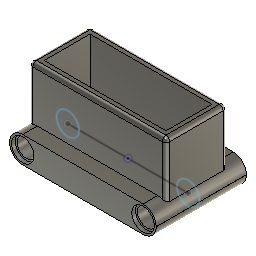
Servo_mount (Autodesk Fusion 360 design; units mm, degrees)
Autodesk Fusion 360 part; units mm, degrees
note: some values were not read from the file. Set by a fixed rule: which face or edge a step refers to.
sketch "Sketch1" plane through (0, 0, 0) normal (0, 1, 0) x (1, 0, 0)
  circle A0 centre (-16, 0) radius 2.5
  circle A1 centre (16, 0) radius 2.5
  line L0 (16.01, -3.5) -> (-16.01, -3.5)
  line L1 (-19.5, -0.01) -> (-19.5, 0.01)
  line L2 (-16.01, 3.5) -> (16.01, 3.5)
  line L3 (19.5, 0.01) -> (19.5, -0.01)
  arc A2 (-16.01, 3.5) -> (-19.5, 0.01) centre (-16.01, 0.01) ccw
  arc A3 (-19.5, -0.01) -> (-16.01, -3.5) centre (-16.01, -0.01) ccw
  arc A4 (19.5, 0.01) -> (16.01, 3.5) centre (16.01, 0.01) ccw
  arc A5 (16.01, -3.5) -> (19.5, -0.01) centre (16.01, -0.01) ccw
  line L4 (-13.5, 0) -> (-16, 0)
  circle A6 centre (16.01, 0.01) radius 3
  circle A7 centre (-16, 0) radius 3
  dimension "d7" = 5
  dimension "d9" = 5
  dimension "d12" = 3.49
  dimension "d13" = 3.49
  dimension "d14" = 3.49
  dimension "d15" = 3.49
  dimension "d53" = 6
  dimension "d54" = 6
  constraint coincident A0.centre L4.end
  constraint horizontal L0
  constraint perpendicular L0 L1
  constraint parallel L0 L2
  constraint parallel L1 L3
  constraint tangent L2 A2
  constraint tangent L1 A2
  constraint tangent L1 A3
  constraint tangent L0 A3
  constraint tangent L2 A4
  constraint tangent L3 A4
  constraint tangent L0 A5
  constraint tangent L3 A5
  constraint coincident A0 L4.start
  constraint concentric A4 A6
  measures "d7" diameter of A0
  measures "d9" diameter of A1
  measures "d12" radius of A2
  measures "d13" radius of A3
  measures "d14" radius of A4
  measures "d15" radius of A5
  measures "d53" diameter of A6
  measures "d54" diameter of A7
sketch "Sketch2" plane through (0, 0, 0) normal (0, 0, 1) x (1, 0, 0)
  line L0 (16.2, 6.1) -> (-16.2, 6.1)
  line L1 (-16.2, 6.1) -> (-16.2, -6.1)
  line L2 (-16.2, -6.1) -> (16.2, -6.1)
  line L3 (16.2, -6.1) -> (16.2, 6.1)
  line L4 (16.2, 6.1) -> (-16.2, -6.1) construction
  line L5 (-16.2, 6.1) -> (16.2, -6.1) construction
  line L6 (11.5, 6.1) -> (-11.5, 6.1)
  line L7 (-11.5, 6.1) -> (-11.5, -6.1)
  line L8 (-11.5, -6.1) -> (11.5, -6.1)
  line L9 (11.5, -6.1) -> (11.5, 6.1)
  line L10 (11.5, 6.1) -> (-11.5, -6.1) construction
  line L11 (-11.5, 6.1) -> (11.5, -6.1) construction
  line L12 (0, 0) -> (14, 0)
  line L13 (0, 0) -> (-14, 0)
  circle A0 centre (14, 0) radius 0.75
  circle A1 centre (-14, 0) radius 0.75
  line L14 (18.2, -8.1) -> (-18.2, -8.1)
  line L15 (-18.2, -8.1) -> (-18.2, 8.1)
  line L16 (-18.2, 8.1) -> (18.2, 8.1)
  line L17 (18.2, 8.1) -> (18.2, -8.1)
  line L18 (18.2, -8.1) -> (-18.2, 8.1) construction
  line L19 (-18.2, -8.1) -> (18.2, 8.1) construction
  dimension "d16" = 32.4
  dimension "d17" = 12.2
  dimension "d18" = 23
  dimension "d19" = 14
  dimension "d20" = 14
  dimension "d21" = 1.5
  dimension "d22" = 1.5
  dimension "d23" = 36.4
  dimension "d24" = 16.2
  constraint horizontal L0
  constraint perpendicular L0 L1
  constraint parallel L0 L2
  constraint parallel L1 L3
  constraint coincident L4 L12.start
  constraint coincident L5 L12.start
  constraint coincident L12.start L13.start
  constraint horizontal L6
  constraint perpendicular L6 L7
  constraint parallel L6 L8
  constraint parallel L7 L9
  constraint coincident L10 L12.start
  constraint coincident L11 L12.start
  constraint horizontal L12
  constraint horizontal L13
  constraint coincident L12.end A0.centre
  constraint coincident L13.end A1.centre
  constraint horizontal L14
  constraint perpendicular L14 L15
  constraint parallel L14 L16
  constraint parallel L15 L17
  constraint coincident L18 L12.start
  constraint coincident L19 L12.start
  measures "d16" distance of L1.end L2.end
  measures "d17" distance of L0.end L1.end
  measures "d18" distance of L7.end L8.end
  measures "d19" distance of L12.start L12.end
  measures "d20" distance of L12.start L13.end
  measures "d21" diameter of A0
  measures "d22" diameter of A1
  measures "d23" distance of L15.end L16.end
  measures "d24" distance of L14.end L15.end
extrude "Extrude1" add sketch "Sketch2" along normal blind 7 contours L14 L15 L16 L17
extrude "Extrude2" add sketch "Sketch2" along normal blind 4 contours L0 L2 L3 L9 | L0 L1 L2 L7
move_body "Move1" bodies 1 to x (1, 0, 0) y (0, 1, 0) z (0, 0, 1) at (0, 0, 0.5)
extrude "Extrude3" cut sketch "Sketch1" along normal blind 9 contours A0 | A1
extrude "Extrude4" cut sketch "Sketch1" against normal blind 10 contours A0 | A1
extrude "Extrude5" add sketch "Sketch1" along normal blind 12 contours L0 L1 L2 L3 A2 A3 A4 A5 | A6 | A7
extrude "Extrude6" add sketch "Sketch1" against normal blind 12 contours L0 L1 L2 L3 A2 A3 A4 A5 | A6 | A7
extrude "Extrude7" cut 4 faces at (-14.1944, 0.2437, 3.5) (-13.8167, -0.17, 3.5) (14.2094, 0.1781, 3.5) (14.1587, -0.2327, 3.5) along direction (0, 0, -1) blind 6
extrude "Extrude8" cut 1 faces at (-3.8333, 2.0333, 3.5) along direction (0, 0, -1) blind 100
sketch "Sketch3" plane through (0, -12, 0) normal (0, -1, 0) x (1, 0, 0)
  circle A0 centre (16, 0) radius 2.5
  circle A1 centre (-16, 0) radius 2.5
  arc A2 (-16.01, 3.5) -> (-19.5, 0.01) centre (-16.01, 0.01) ccw
  line L0 (-19.5, 0.01) -> (-19.5, -0.01)
  arc A3 (-19.5, -0.01) -> (-16.01, -3.5) centre (-16.01, -0.01) ccw
  line L1 (-16.01, -3.5) -> (16.01, -3.5)
  arc A4 (16.01, -3.5) -> (19.5, -0.01) centre (16.01, -0.01) ccw
  line L2 (19.5, -0.01) -> (19.5, 0.01)
  arc A5 (19.5, 0.01) -> (16.01, 3.5) centre (16.01, 0.01) ccw
  line L3 (16.01, 3.5) -> (-16.01, 3.5)
  circle A6 centre (-16, 0) radius 3
  circle A7 centre (16, 0) radius 3
  dimension "d41" = 6
  dimension "d42" = 6
  constraint concentric A1 A6
  constraint concentric A0 A7
  measures "d41" diameter of A6
  measures "d42" diameter of A7
extrude "Extrude9" cut sketch "Sketch3" against normal blind 1 contours A6
extrude "Extrude10" cut sketch "Sketch3" against normal blind 1 contours A7
sketch "Sketch4" plane through (0, 12, 0) normal (0, 1, 0) x (-1, 0, 0)
  circle A0 centre (16, 0) radius 2.5
  circle A1 centre (-16, 0) radius 2.5
  arc A2 (19.5, 0.01) -> (16.01, 3.5) centre (16.01, 0.01) ccw
  line L0 (16.01, 3.5) -> (-16.01, 3.5)
  arc A3 (-16.01, 3.5) -> (-19.5, 0.01) centre (-16.01, 0.01) ccw
  line L1 (-19.5, 0.01) -> (-19.5, -0.01)
  arc A4 (-19.5, -0.01) -> (-16.01, -3.5) centre (-16.01, -0.01) ccw
  line L2 (-16.01, -3.5) -> (16.01, -3.5)
  arc A5 (16.01, -3.5) -> (19.5, -0.01) centre (16.01, -0.01) ccw
  line L3 (19.5, -0.01) -> (19.5, 0.01)
  circle A6 centre (-16, 0) radius 3
  circle A7 centre (16, 0) radius 3
  dimension "d47" = 6
  dimension "d48" = 6
  constraint concentric A1 A6
  constraint concentric A0 A7
  measures "d47" diameter of A6
  measures "d48" diameter of A7
extrude "Extrude11" cut sketch "Sketch4" against normal blind 1 contours A6
extrude "Extrude12" cut sketch "Sketch4" against normal blind 1 contours A7
sketch "Sketch5" plane through (0, 0, 0) normal (0, 1, 0) x (1, 0, 0)
  line L0 (0, 0) -> (16, 0)
  line L1 (0, 0) -> (-16, 0)
  circle A0 centre (-16, 0) radius 3
  circle A1 centre (16, 0) radius 3
  dimension "d55" = 6
  dimension "d56" = 6
  constraint coincident L0.start L1.start
  constraint horizontal L0
  constraint parallel L0 L1
  constraint coincident L1.end A0.centre
  constraint coincident L0.end A1.centre
  measures "d55" diameter of A0
  measures "d56" diameter of A1
extrude "Extrude13" cut sketch "Sketch5" against normal blind 5 contours A0
extrude "Extrude14" cut sketch "Sketch5" along normal blind 5 contours A0
extrude "Extrude15" cut sketch "Sketch5" along normal blind 5 contours A1
extrude "Extrude16" cut sketch "Sketch5" against normal blind 5 contours A1
extrude "Extrude17" add 1 faces at (5.4, -7.4333, 7.5) along direction (0, 0, 1) blind 10
fillet "Fillet1" radius 1 8 edges at (-18.2, 8.1, 10.1137) (-18.2, -8.1, 10.1137) (18.2, -8.1, 10.1137) (18.2, 8.1, 10.1137) (18.2, 0, 17.5) (0, 8.1, 17.5) (0, -8.1, 17.5) (-18.2, 0, 17.5)
